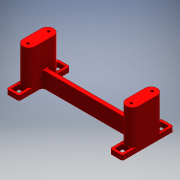
# Autodesk Inventor part: red_part
Saved by Autodesk Inventor 2016 (Build 200138000, 138)
## iProperties
Created: 2016-07-26
Part Number: red_part
Material: Plastique ABS
Document SubType Name: Modeling
Designer: tmonglon
Density: 1.06 g/cm^3
Appearance: Lisse - Rouge
Author: tmonglon
Autodesk Inventor part; units mm, degrees
ref_plane "YZ Plane" through (0, 0, 0) normal (1, 0, 0) x (0, 1, 0)
ref_plane "XZ Plane" through (0, 0, 0) normal (0, 1, 0) x (-1, 0, 0)
ref_plane "XY Plane" through (0, 0, 0) normal (0, 0, 1) x (1, 0, 0)
sketch "Esquisse1" plane through (0, 0, 0) normal (0, 0, 1) x (1, 0, 0)
  line L0 (75, 0) -> (75, 33)
  line L1 (0, 33) -> (0, 0)
  line L2 (8, 33) -> (8, 0)
  line L3 (67, 33) -> (67, 0)
  line L4 (8, 17.75) -> (67, 17.75)
  line L5 (67, 17.75) -> (67, 15.25)
  line L6 (67, 15.25) -> (8, 15.25)
  line L7 (8, 15.25) -> (8, 17.75)
  line L8 (75, 33) -> (67, 33)
  line L9 (8, 33) -> (0, 33)
  line L10 (0, 0) -> (8, 0)
  line L11 (67, 0) -> (75, 0)
  line L12 (1.5, 6.5) -> (6.5, 6.5)
  line L13 (6.5, 6.5) -> (6.5, 1.5)
  line L14 (6.5, 1.5) -> (1.5, 1.5)
  line L15 (1.5, 1.5) -> (1.5, 6.5)
  line L16 (0, 16.5) -> (-2.6312, 16.5)
  line L17 (37.5, 15.25) -> (37.5, 13.3261)
  line L18 (1.5, 26.5) -> (6.5, 26.5)
  line L19 (6.5, 26.5) -> (6.5, 31.5)
  line L20 (6.5, 31.5) -> (1.5, 31.5)
  line L21 (1.5, 31.5) -> (1.5, 26.5)
  line L22 (73.5, 6.5) -> (68.5, 6.5)
  line L23 (68.5, 6.5) -> (68.5, 1.5)
  line L24 (68.5, 1.5) -> (73.5, 1.5)
  line L25 (73.5, 1.5) -> (73.5, 6.5)
  line L26 (68.5, 26.5) -> (68.5, 31.5)
  line L27 (68.5, 31.5) -> (73.5, 31.5)
  line L28 (73.5, 31.5) -> (73.5, 26.5)
  line L29 (73.5, 26.5) -> (68.5, 26.5)
  arc A0 (8, 22.5) -> (0, 22.5) centre (4, 22.5) ccw
  arc A1 (0, 10.5) -> (8, 10.5) centre (4, 10.5) ccw
  arc A2 (75, 22.5) -> (67, 22.5) centre (71, 22.5) ccw
  arc A3 (67, 10.5) -> (75, 10.5) centre (71, 10.5) ccw
  line L30 (67, 22.5) -> (67, 10.5)
  line L31 (75, 10.5) -> (75, 22.5)
  line L32 (8, 22.5) -> (8, 10.5)
  line L33 (0, 10.5) -> (0, 22.5)
  dimension "d0" = 33
  dimension "d1" = 75
  dimension "d2" = 8
  dimension "d3" = 8
  dimension "d4" = 2.5
  dimension "d6" = 5
  dimension "d7" = 5
  dimension "d8" = 1.5
  dimension "d9" = 1.5
  dimension "d10" = 8
  dimension "d11" = 8
  dimension "d12" = 12
  dimension "d13" = 10.5
  constraints: 68 end point, 14 symmetric about line, 10 parallel, 10 point on line, 8 perpendicular, 8 point on circle, 5 horizontal, 4 centre point, 3 collinear, 3 tangent, 2 midpoint, 1 vertical, 2 other
  measures "d0" distance of L1.start L1.end
  measures "d1" distance of L1.end L0.start
  measures "d2" distance between parallel lines of L2 L1
  measures "d3" distance between parallel lines of L0 L3
  measures "d4" distance between parallel lines of L6 L4
  measures "d6" distance of L13.end L14.end
  measures "d7" distance of L14.end L12.start
  measures "d8" distance between parallel lines of L10 L14
  measures "d9" distance between parallel lines of L1 L15
  measures "d10" diameter of A0
  measures "d11" diameter of A1
  measures "d12" distance of A1.centre A0.centre
  measures "d13" distance from line of L9 A0.centre
extrude "Extrusion1" add sketch "Esquisse1" along normal blind 3 contours L11 L3 A3 L0 | A2 L3 L8 L0 | A0 L1 L9 L2 | L2 L10 L1 A1
extrude "Extrusion2" add sketch "Esquisse1" along normal blind 25.5 contours A3 L3 A2 L0 | L2 A1 L1 A0
extrude "Extrusion3" add sketch "Esquisse1" along normal blind 10 contours L6 L2 L4 L3
fillet "Congé1" radius 2 4 edges at (8, 15.25, 5) (8, 17.75, 5) (67, 15.25, 5) (67, 17.75, 5)
hole "Perçage1" at (71, 23.25, 25.5) direction (0, 0, -1) diameter 1.6 depth 10 tip angle 118
hole "Perçage2" at (71, 9.75, 25.5) direction (0, 0, -1) diameter 1.6 depth 10 tip angle 118
hole "Perçage3" at (4, 23.25, 25.5) direction (0, 0, -1) diameter 1.6 depth 10 tip angle 118
hole "Perçage4" at (4, 9.75, 25.5) direction (0, 0, -1) diameter 1.6 depth 10 tip angle 118
fillet "Congé2" radius 1 8 edges at (8, 0, 1.5) (0, 0, 1.5) (67, 0, 1.5) (75, 0, 1.5) (67, 33, 1.5) (75, 33, 1.5) (8, 33, 1.5) (0, 33, 1.5)
equation "\"d9\" = -0.5 * d6 + 0.5 * d2"
equation "\"d13\" = -0.5 * d12 + 0.5 * d0"
